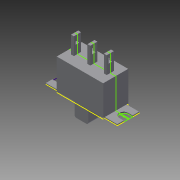
# Autodesk Inventor part: Power_Switch
Saved by Autodesk Inventor 2015 (Build 190159000, 159)
## iProperties
Created: 2014-12-09
Part Number: Power_Switch
Material: Generic
Document SubType Name: Modeling
Designer: Temp2
Density: 1 g/cm^3
Appearance: Default
Author: Temp2
Autodesk Inventor part; units mm, degrees
ref_plane "YZ Plane" through (0, 0, 0) normal (1, 0, 0) x (0, 1, 0)
ref_plane "XZ Plane" through (0, 0, 0) normal (0, 1, 0) x (-1, 0, 0)
ref_plane "XY Plane" through (0, 0, 0) normal (0, 0, 1) x (1, 0, 0)
sketch "Sketch1" plane through (0, 0, 0) normal (0, 1, 0) x (-1, 0, 0)
  line L0 (10, 0.3) -> (-10, 0.3)
  line L1 (-10, 0.3) -> (-10, 0)
  line L2 (-10, 0) -> (10, 0)
  line L3 (10, 0) -> (10, 0.3)
  line L4 (-6.5, 0.3) -> (6.5, 0.3)
  line L5 (6.5, 0.3) -> (6.5, 8.7)
  line L6 (6.5, 8.7) -> (-6.5, 8.7)
  line L7 (-6.5, 8.7) -> (-6.5, 0.3)
  line L8 (6.5, 8.7) -> (5, 8.7)
  line L9 (0.4, 8.7) -> (0.4, 13.5)
  line L10 (-0.4, 13.5) -> (-0.4, 8.7)
  line L11 (-4.2, 13.5) -> (-4.2, 8.7)
  line L12 (-5, 8.7) -> (-5, 13.5)
  line L13 (4.2, 13.5) -> (4.2, 8.7)
  line L14 (5, 8.7) -> (5, 13.5)
  line L15 (4.2, 13.5) -> (5, 13.5)
  line L16 (-5, 13.5) -> (-4.2, 13.5)
  line L17 (-0.4, 13.5) -> (0.4, 13.5)
  line L18 (4.2, 8.7) -> (-6.5, 8.7)
  line L19 (5, 8.7) -> (4.2, 8.7)
  point P0 (0, 0)
  point P1 (0, 0)
  dimension "d0" = 20
  dimension "d1" = 0.3
  dimension "d2" = 13
  dimension "d6" = 8.7
  dimension "d7" = 13.5
  constraints: 40 end point, 14 perpendicular, 13 parallel, 9 point on line, 5 horizontal, 1 midpoint
  measures "d0" distance of L2.end L1.end
  measures "d1" distance of L1.end L0.end
  measures "d2" distance of L6.end L5.end
  measures "d6" distance between parallel lines of L8 L2
  measures "d7" distance between parallel lines of L15 L2
extrude "Extrusion1" add sketch "Sketch1" along normal mid plane 7 contours L0 L7 L6 L5
extrude "Extrusion2" add sketch "Sketch1" along normal mid plane 6.1 contours L3 L2 L1 L0
extrude "Extrusion3" add sketch "Sketch1" along normal mid plane 2 contours L6 L13 L15 L14 | L12 L16 L11 L6 | L6 L10 L17 L9
sketch "Sketch2" plane through (10, 3.05, 0) normal (0, 0, -1) x (-1, 0, 0)
  line L0 (0, -6.1) -> (0, 0) projected
  line L1 (20, -6.1) -> (20, 0) projected
  line L2 (20, -6.1) -> (0, -6.1) projected
  line L3 (0, 0) -> (20, 0) projected
  arc A0 (18.75, -1.8) -> (18.75, -4.3) centre (18.75, -3.05) ccw
  line L4 (18.75, -4.3) -> (20, -4.3)
  line L5 (18.75, -1.8) -> (20, -1.8)
  arc A1 (1.25, -4.3) -> (1.25, -1.8) centre (1.25, -3.05) ccw
  line L6 (1.25, -4.3) -> (0, -4.3)
  line L7 (1.25, -1.8) -> (0, -1.8)
  line L8 (13.05, -1.1) -> (6.95, -1.1)
  line L9 (6.95, -1.1) -> (6.95, -5)
  line L10 (6.95, -5) -> (13.05, -5)
  line L11 (13.05, -5) -> (13.05, -1.1)
  line L12 (13.05, -1.1) -> (9.25, -1.1)
  line L13 (9.25, -1.1) -> (9.25, -5)
  line L14 (9.25, -5) -> (13.05, -5)
  line L15 (13.05, -5) -> (13.05, -1.1)
  line L16 (0, -1.8) -> (0, -4.3)
  line L17 (20, -1.8) -> (20, -4.3)
  line L18 (3.5, 0.45) -> (16.5, 0.45) projected
  line L19 (16.5, -6.55) -> (3.5, -6.55) projected
  point P0 (10, -3.05)
  dimension "d16" = 6.1
  dimension "d17" = 2.5
  dimension "d18" = 17.5
  dimension "d22" = 3.9
  dimension "d23" = 6.1
  dimension "d24" = 3.8
  dimension "d34" = 7
  constraints: 28 end point, 4 parallel, 4 point on circle, 3 horizontal, 3 perpendicular, 3 point on line, 2 centre point, 2 tangent, 1 collinear, 1 vertical
  measures "d16" distance between parallel lines of L2 L3
  measures "d17" diameter of A0
  measures "d18" distance of A1.centre A0.centre
  measures "d22" distance of L9.end L8.end
  measures "d23" distance between parallel lines of L9 L11
  measures "d24" distance of L14.end L13.end
  measures "d34" distance between parallel lines of L18 L19
extrude "Extrusion4" cut sketch "Sketch2" against normal blind 0.3 contours L0 L7 A1 L6 | L4 A0 L5 L1
extrude "Extrusion5" add sketch "Sketch2" along normal blind 5 contours L11 L10 L13 L8
fillet "Fillet1" radius 0.5 2 edges at (0.75, 0, -5) (-3.05, 0, -5)
sketch "Sketch3" plane through (-5, -1, 13.5) normal (-1, 0, 0) x (0, 0, 1)
  line L0 (-0.5, 0.5) -> (-2.3, 0.5)
  line L1 (-2.3, 0.5) -> (-2.3, 1.5)
  line L2 (-2.3, 1.5) -> (-0.5, 1.5)
  line L3 (-0.5, 1.5) -> (-0.5, 0.5)
  point P0 (-13.5, 1)
  dimension "d30" = 1.8
  dimension "d31" = 1
  constraints: 8 end point, 2 parallel, 1 horizontal, 1 perpendicular
  measures "d30" distance of L1.end L2.end
  measures "d31" distance of L0.end L1.end
extrude "Extrusion6" cut sketch "Sketch3" against normal blind 13
body "Solid1"
